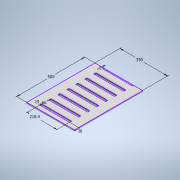
# Autodesk Inventor part: end_part_ferrite
Saved by Autodesk Inventor 2020 (Build 240168000, 168)
## iProperties
Created: 2021-01-27
Part Number: end_part_ferrite
Material: Generic
Document SubType Name: Modeling
Designer: apat475
Density: 1 g/cm^3
Appearance: Default
Author: apat475
Autodesk Inventor part; units mm, degrees
ref_plane "YZ Plane" through (0, 0, 0) normal (1, 0, 0) x (0, 1, 0)
ref_plane "XZ Plane" through (0, 0, 0) normal (0, 1, 0) x (-1, 0, 0)
ref_plane "XY Plane" through (0, 0, 0) normal (0, 0, 1) x (1, 0, 0)
sketch "Sketch1" plane through (0, 0, 0) normal (0, 1, 0) x (-1, 0, 0)
  line L0 (93.9879, 313.0349) -> (-256.0121, 313.0349)
  line L1 (-256.0121, 313.0349) -> (-256.0121, -186.9651)
  line L2 (-256.0121, -186.9651) -> (93.9879, -186.9651)
  line L3 (93.9879, -186.9651) -> (93.9879, 313.0349)
  line L4 (27.9879, 283.0349) -> (-190.4121, 283.0349)
  line L5 (-190.4121, 283.0349) -> (-190.4121, 268.0349)
  line L6 (-190.4121, 268.0349) -> (27.9879, 268.0349)
  line L7 (27.9879, 268.0349) -> (27.9879, 283.0349)
  line L8 (27.9879, 217.0349) -> (-190.4121, 217.0349)
  line L9 (-190.4121, 217.0349) -> (-190.4121, 202.0349)
  line L10 (-190.4121, 202.0349) -> (27.9879, 202.0349)
  line L11 (27.9879, 202.0349) -> (27.9879, 217.0349)
  line L12 (27.9879, 151.0349) -> (-190.4121, 151.0349)
  line L13 (-190.4121, 151.0349) -> (-190.4121, 136.0349)
  line L14 (-190.4121, 136.0349) -> (27.9879, 136.0349)
  line L15 (27.9879, 136.0349) -> (27.9879, 151.0349)
  line L16 (27.9879, 85.0349) -> (-190.4121, 85.0349)
  line L17 (-190.4121, 85.0349) -> (-190.4121, 70.0349)
  line L18 (-190.4121, 70.0349) -> (27.9879, 70.0349)
  line L19 (27.9879, 70.0349) -> (27.9879, 85.0349)
  line L20 (27.9879, 19.0349) -> (-190.4121, 19.0349)
  line L21 (-190.4121, 19.0349) -> (-190.4121, 4.0349)
  line L22 (-190.4121, 4.0349) -> (27.9879, 4.0349)
  line L23 (27.9879, 4.0349) -> (27.9879, 19.0349)
  line L24 (27.9879, -46.9651) -> (-190.4121, -46.9651)
  line L25 (-190.4121, -46.9651) -> (-190.4121, -61.9651)
  line L26 (-190.4121, -61.9651) -> (27.9879, -61.9651)
  line L27 (27.9879, -61.9651) -> (27.9879, -46.9651)
  line L28 (27.9879, -112.9651) -> (-190.4121, -112.9651)
  line L29 (-190.4121, -112.9651) -> (-190.4121, -127.9651)
  line L30 (-190.4121, -127.9651) -> (27.9879, -127.9651)
  line L31 (27.9879, -127.9651) -> (27.9879, -112.9651)
  line L32 (27.9879, -186.9651) -> (27.9879, -178.9651)
  line L33 (27.9879, -178.9651) -> (-190.0121, -178.9651)
  line L34 (-190.0121, -178.9651) -> (-190.0121, -186.9651)
  dimension "d0" = 500
  dimension "d1" = 350
  dimension "d11" = 15
  dimension "d13" = 30
  dimension "d22" = 66
  dimension "d27" = 8
  dimension "d28" = 218.4
  constraints: 70 end point, 5 perpendicular, 4 parallel, 2 horizontal, 2 point on line, 1 vertical, 48 other
  measures "d0" distance of L2.end L0.start
  measures "d1" distance of L1.end L2.end
  measures "d11" distance of L6.end L4.start
  measures "d13" distance between parallel lines of L0 L4
  measures "d22" distance of L4.start L8.start
  measures "d27" distance of L32.start L32.end
  measures "d28" distance of L4.start L4.end
extrude "Extrusion2" add sketch "Sketch1" against normal blind 8 contours L3 L2 L32 L33 L34 L1 L0 | L2 L34 L33 L32 | L11 L10 L9 L8 | L15 L14 L13 L12 | L19 L18 L17 L16 | L23 L22 L21 L20 | L27 L26 L25 L24 | L31 L30 L29 L28
extrude "Extrusion3" cut sketch "Sketch1" against normal up to surface (8 mm away) contours L11 L10 L9 L8 | L15 L14 L13 L12 | L19 L18 L17 L16 | L23 L22 L21 L20 | L27 L26 L25 L24 | L31 L30 L29 L28
extrude "Extrusion4" cut sketch "Sketch1" against normal up to surface (8 mm away) contours L2 L34 L33 L32
body "Solid2"
